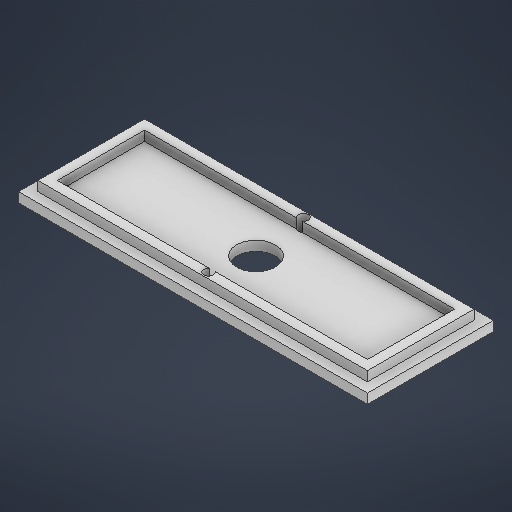
# Autodesk Inventor part: five_cell_top_case
Saved by Autodesk Inventor 2026 (Build 300175050, 175E)
## iProperties
Created: 2025-06-13
Part Number: five_cell_top_case
Material: Generic
Document SubType Name: Modeling
Designer: hamth
Density: 1 g/cm^3
Appearance: Default
Author: hamth
Autodesk Inventor part; units mm, degrees
ref_plane "YZ Plane" through (0, 0, 0) normal (1, 0, 0) x (0, 1, 0)
ref_plane "XZ Plane" through (0, 0, 0) normal (0, 1, 0) x (-1, 0, 0)
ref_plane "XY Plane" through (0, 0, 0) normal (0, 0, 1) x (1, 0, 0)
sketch "Sketch1" plane through (0, 0, 0) normal (0, 1, 0) x (-1, 0, 0)
  line L0 (74.4424, -50.7093) -> (-39.8576, -50.7093)
  line L1 (-39.8576, -50.7093) -> (-39.8576, -9.4343)
  line L2 (-39.8576, -9.4343) -> (74.4424, -9.4343)
  line L3 (74.4424, -9.4343) -> (74.4424, -50.7093)
  point P0 (0, 0)
  dimension "d0" = 41.275
  dimension "d1" = 114.3
  constraints: 8 end point, 2 parallel, 1 horizontal, 1 perpendicular
  measures "d0" distance of L2.end L0.start
  measures "d1" distance of L0.start L0.end
extrude "Extrusion1" add sketch "Sketch1" along normal blind 3.175
sketch "Sketch2" plane through (0, 3.175, 0) normal (0, 1, 0) x (1, 0, 0)
  line L0 (-74.4424, 50.7093) -> (-74.4424, 9.4343) projected
  line L1 (-74.4424, 50.7093) -> (-71.2674, 50.7093)
  line L2 (39.8576, 50.7093) -> (-74.4424, 50.7093) projected
  line L3 (-71.2674, 50.7093) -> (-71.2674, 47.5343)
  line L4 (-71.2674, 47.5343) -> (-68.0924, 47.5343)
  line L5 (-68.0924, 47.5343) -> (-68.0924, 12.6093)
  line L6 (-68.0924, 12.6093) -> (-71.2674, 12.6093)
  line L7 (-71.2674, 12.6093) -> (-71.2674, 47.5343)
  point P0 (0, 0)
  dimension "d4" = 3.175
  dimension "d5" = 3.175
  dimension "d6" = 3.175
  dimension "d7" = 34.925
  constraints: 12 end point, 2 parallel, 1 horizontal, 1 perpendicular, 1 point on line, 1 vertical
  measures "d4" distance of L0.start L1.end
  measures "d5" distance of L1.end L3.end
  measures "d6" distance of L3.end L4.end
  measures "d7" distance of L4.end L5.end
extrude "Extrusion2" add sketch "Sketch2" along normal blind 3.175
sketch "Sketch3" plane through (0, 3.175, 0) normal (0, 1, 0) x (1, 0, 0)
  line L0 (39.8576, 9.4343) -> (39.8576, 50.7093) projected
  line L1 (39.8576, 50.7093) -> (36.6826, 50.7093)
  line L2 (39.8576, 50.7093) -> (-74.4424, 50.7093) projected
  line L3 (36.6826, 50.7093) -> (36.6826, 47.5343)
  line L4 (36.6826, 47.5343) -> (33.5076, 47.5343)
  line L5 (33.5076, 47.5343) -> (33.5076, 12.6093)
  line L6 (33.5076, 12.6093) -> (36.6826, 12.6093)
  line L7 (36.6826, 12.6093) -> (36.6826, 47.5343)
  point P0 (0, 0)
  dimension "d10" = 3.175
  dimension "d11" = 3.175
  dimension "d12" = 3.175
  dimension "d13" = 34.925
  constraints: 12 end point, 2 parallel, 1 horizontal, 1 perpendicular, 1 point on line, 1 vertical
  measures "d10" distance of L0.end L1.end
  measures "d11" distance of L1.end L3.end
  measures "d12" distance of L5.end L6.end
  measures "d13" distance of L4.end L5.end
extrude "Extrusion3" add sketch "Sketch3" along normal blind 3.175
sketch "Sketch4" plane through (0, 3.175, 0) normal (0, 1, 0) x (1, 0, 0)
  line L0 (-68.0924, 47.5343) -> (-68.0924, 12.6093) projected
  line L1 (-68.0924, 47.5343) -> (33.5076, 47.5343)
  line L2 (33.5076, 47.5343) -> (33.5076, 44.3593)
  line L3 (33.5076, 44.3593) -> (-68.0924, 44.3593)
  line L4 (-68.0924, 44.3593) -> (-68.0924, 47.5343)
  point P0 (0, 0)
  dimension "d16" = 3.175
  dimension "d17" = 101.6
  constraints: 8 end point, 2 parallel, 1 horizontal, 1 perpendicular
  measures "d16" distance of L1.end L2.end
  measures "d17" distance of L2.end L3.end
extrude "Extrusion4" add sketch "Sketch4" along normal blind 3.175
sketch "Sketch5" plane through (0, 3.175, 0) normal (0, 1, 0) x (1, 0, 0)
  line L0 (-71.2674, 12.6093) -> (-68.0924, 12.6093) projected
  line L1 (-68.0924, 12.6093) -> (33.5076, 12.6093)
  line L2 (33.5076, 12.6093) -> (33.5076, 15.7843)
  line L3 (33.5076, 15.7843) -> (-68.0924, 15.7843)
  line L4 (-68.0924, 15.7843) -> (-68.0924, 12.6093)
  point P0 (0, 0)
  dimension "d20" = 3.175
  dimension "d21" = 101.6
  constraints: 8 end point, 2 parallel, 1 horizontal, 1 perpendicular
  measures "d20" distance of L1.end L2.end
  measures "d21" distance of L2.end L3.end
extrude "Extrusion5" add sketch "Sketch5" along normal blind 3.175
sketch "Sketch10" plane through (0, 0, 0) normal (0, -1, 0) x (1, 0, 0)
  line L0 (39.8576, -9.4343) -> (39.8576, -30.0718)
  line L1 (39.8576, -9.4343) -> (39.8576, -50.7093) projected
  line L2 (39.8576, -30.0718) -> (-17.2924, -30.0718)
  point P0 (0, 0)
  dimension "d38" = 20.6375
  dimension "d39" = 57.15
  constraints: 4 end point, 1 midpoint, 1 perpendicular
  measures "d38" distance of L0.start L0.end
  measures "d39" distance of L0.end L2.end
hole "Hole2" at (-17.2924, 0, -30.0718) direction (0, 1, 0) diameter 12.7 end through all
sketch "Sketch13" plane through (0, 0, 0) normal (0, -1, 0) x (1, 0, 0)
  line L0 (39.8576, -9.4343) -> (39.8576, -50.7093) projected
  line L1 (39.8576, -9.4343) -> (39.8576, -14.5143)
  line L2 (39.8576, -14.5143) -> (-17.2924, -14.5143)
  point P0 (0, 0)
  dimension "d51" = 5.08
  dimension "d52" = 57.15
  constraints: 4 end point, 1 perpendicular, 1 point on line
  measures "d51" distance of L0.start L1.end
  measures "d52" distance of L1.end L2.end
hole "Hole3" at (-17.2924, 0, -14.5143) direction (0, 1, 0) diameter 3.175 end through all
sketch "Sketch14" plane through (0, 0, 0) normal (0, -1, 0) x (1, 0, 0)
  line L0 (39.8576, -9.4343) -> (39.8576, -50.7093) projected
  line L1 (39.8576, -50.7093) -> (39.8576, -45.6293)
  line L2 (39.8576, -45.6293) -> (-17.2924, -45.6293)
  point P0 (0, 0)
  dimension "d60" = 5.08
  dimension "d61" = 57.15
  constraints: 4 end point, 1 perpendicular, 1 point on line
  measures "d60" distance of L0.end L1.end
  measures "d61" distance of L1.end L2.end
hole "Hole4" at (-17.2924, 0, -45.6293) direction (0, 1, 0) diameter 3.175 end through all
body "Solid1"
